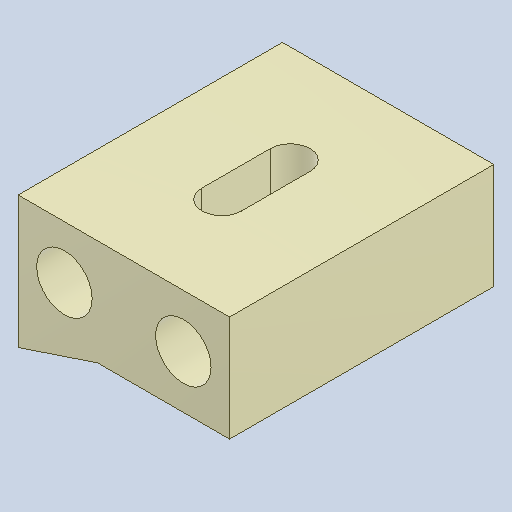
# Autodesk Inventor part: стена_каретки
Saved by Autodesk Inventor 2023.1 (Build 271208000, 208)
## iProperties
Created: 2026-01-04
Part Number: стена_каретки
Material: Полипропилен
Document SubType Name: Modeling
Designer: DELL
Density: 0.899 g/cm^3
Appearance: Гладкий — пепельный
Author: DELL
Autodesk Inventor part; units mm, degrees
ref_plane "YZ Plane" through (0, 0, 0) normal (1, 0, 0) x (0, 1, 0)
ref_plane "XZ Plane" through (0, 0, 0) normal (0, 1, 0) x (-1, 0, 0)
ref_plane "XY Plane" through (0, 0, 0) normal (0, 0, 1) x (1, 0, 0)
sketch "Эскиз1" plane through (0, 0, 0) normal (0, 0, 1) x (1, 0, 0)
  line L0 (13.5, 19.05) -> (-13.5, 19.05) construction
  circle A0 centre (-7.5, -8) radius 1.6 construction
  circle A1 centre (7.5, -8) radius 1.6 construction
  line L1 (-13.5, 19.05) -> (2.5, 19.05)
  line L2 (-13.5, 19.05) -> (-13.5, 9.05)
  line L3 (-7.5, 11.05) -> (2.5, 11.05)
  line L4 (-7.5, 11.05) -> (-13.5, 9.05)
  line L5 (2.5, 11.05) -> (2.5, 19.05)
  point P0 (2.5, 15.05)
  dimension "d3" = 6
  dimension "d15" = 16
  constraints: 10 end point, 1 collinear, 1 midpoint, 1 parallel, 1 vertical
  measures "d3" distance from line of L3.start L2
  measures "d15" distance from line of L2 point (2.5, 15.05)
extrude "Выдавливание1" add sketch "Эскиз1" along normal blind 20
ref_plane "РабПлоскость1" through (0, 0, 10) normal (0, 0, -1) x (-1, 0, 0)
sketch "Эскиз4" plane through (0, 0, 20) normal (0, 0, 1) x (1, 0, 0)
  line L0 (2.5, 11.05) -> (2.5, 19.05) construction
  line L1 (2.5, 15.05) -> (-13.5, 15.05) construction
  line L2 (-13.5, 19.05) -> (-13.5, 9.05) construction
  circle A0 centre (-10, 15.05) radius 2.1
  circle A1 centre (-1, 15.05) radius 2.1
  point P0 (0, 0)
  dimension "d16" = 4.2
  dimension "d17" = 4.2
  dimension "d18" = 3.5
  dimension "d19" = 3.5
  constraints: 3 point on line, 2 centre point, 2 end point, 1 horizontal, 1 midpoint
  measures "d16" diameter of A0
  measures "d17" diameter of A1
  measures "d18" distance from line of L0 A1.centre
  measures "d19" distance from line of L2 A0.centre
extrude "Выдавливание4" cut sketch "Эскиз4" against normal blind 5
mirror "Зеркальное отражение2" about plane through (0, 0, 10) normal (0, 0, -1) of "Выдавливание4"
sketch "Эскиз5" plane through (-13.5, 19.05, 0) normal (0, 1, 0) x (1, 0, 0)
  line L0 (16, 0) -> (0, 0) construction
  line L1 (0, 0) -> (0, -20) construction
  line L2 (16, -20) -> (0, -20) construction
  line L3 (16, 0) -> (16, -20) construction
  line L4 (8, -7.407) -> (8, -12.593) construction
  line L5 (6.5, -7.407) -> (6.5, -12.593)
  line L6 (9.5, -12.593) -> (9.5, -7.407)
  arc A0 (9.5, -7.407) -> (6.5, -7.407) centre (8, -7.407) ccw
  arc A1 (6.5, -12.593) -> (9.5, -12.593) centre (8, -12.593) ccw
  point P0 (13.5, 0)
  point P1 (8, -10)
  dimension "d22" = 3
  constraints: 8 end point, 4 point on circle, 4 tangent, 2 centre point, 1 midpoint, 1 parallel, 1 vertical
  measures "d22" diameter of A1
extrude "Выдавливание5" cut sketch "Эскиз5" against normal blind 20
